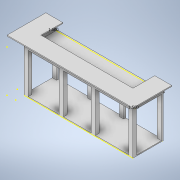
# Autodesk Inventor part: bardraft
Saved by Autodesk Inventor 2020 (Build 240168000, 168)
## iProperties
Created: 2020-07-25
Part Number: bardraft
Material: Generic
Document SubType Name: Modeling
Designer: al
Density: 1 g/cm^3
Appearance: Default
Author: al
Autodesk Inventor part; units mm, degrees
ref_plane "YZ Plane" through (0, 0, 0) normal (1, 0, 0) x (0, 1, 0)
ref_plane "XZ Plane" through (0, 0, 0) normal (0, 1, 0) x (-1, 0, 0)
ref_plane "XY Plane" through (0, 0, 0) normal (0, 0, 1) x (1, 0, 0)
sketch "Sketch1" plane through (0, 0, 0) normal (0, 0, 1) x (1, 0, 0)
  line L0 (0, 0) -> (0, 1092.2)
  line L1 (0, 1092.2) -> (812.8, 1092.2)
  line L2 (812.8, 1092.2) -> (812.8, 0)
  line L3 (812.8, 0) -> (0, 0)
  dimension "d0" = 1092.2
  dimension "d1" = 812.8
  constraints: 8 end point, 3 perpendicular, 1 vertical
  measures "d0" distance of L0.start L0.end
  measures "d1" distance of L0.end L1.end
extrude "Extrusion1" add sketch "Sketch1" along normal blind 2641.6
sketch "Sketch2" plane through (812.8, 0, 0) normal (1, 0, 0) x (0, 0, -1)
  line L0 (-2641.6, 1092.2) -> (-2641.6, 0) projected
  line L1 (-2641.6, 0) -> (-2463.8, 0)
  line L2 (0, 0) -> (-2641.6, 0) projected
  line L3 (-2463.8, 0) -> (-2463.8, 1073.15)
  line L4 (-2463.8, 1073.15) -> (-2641.6, 1073.15)
  line L5 (-2641.6, 1073.15) -> (-2641.6, 0)
  line L6 (0, 1092.2) -> (0, 0) projected
  line L7 (0, 0) -> (-177.8, 0)
  line L8 (-177.8, 0) -> (-177.8, 1073.15)
  line L9 (-177.8, 1073.15) -> (0, 1073.15)
  line L10 (0, 1073.15) -> (0, 0)
  dimension "d4" = 177.8
  dimension "d5" = 1073.15
  dimension "d6" = 177.8
  dimension "d7" = 1073.15
  constraints: 16 end point, 5 perpendicular, 2 point on line, 1 collinear
  measures "d4" distance of L0.end L1.end
  measures "d5" distance of L1.end L3.end
  measures "d6" distance of L2.start L7.end
  measures "d7" distance of L7.end L8.end
extrude "Extrusion2" cut sketch "Sketch2" against normal blind 2641.6
sketch "Sketch3" plane through (812.8, 0, 2463.8) normal (0, 0, 1) x (1, 0, 0)
  line L0 (0, 0) -> (-812.8, 0) projected
  line L1 (-812.8, 0) -> (-635, 0)
  line L2 (-635, 0) -> (-635, 1073.15)
  line L3 (-812.8, 1073.15) -> (0, 1073.15) projected
  line L4 (-812.8, 1073.15) -> (-812.8, 0)
  line L5 (-812.8, 1092.2) -> (-812.8, 1073.15) projected
  line L6 (-635, 1073.15) -> (-812.8, 1073.15)
  dimension "d10" = 177.8
  constraints: 8 end point, 2 point on line, 1 horizontal, 1 parallel, 1 perpendicular
  measures "d10" distance of L0.end L1.end
extrude "Extrusion3" cut sketch "Sketch3" against normal blind 2641.6
sketch "Sketch4" plane through (812.8, 0, 2463.8) normal (0, 0, 1) x (1, 0, 0)
  line L0 (0, 1073.15) -> (0, 0) projected
  line L1 (-635, 1073.15) -> (-635, 0) projected
  line L2 (-635, 0) -> (0, 0) projected
  line L3 (-635, 0) -> (-596.9, 0)
  line L4 (-596.9, 0) -> (-596.9, 19.05)
  line L5 (-596.9, 19.05) -> (-635, 19.05)
  line L6 (0, 0) -> (0, 1073.15) projected
  line L7 (0, 0) -> (0, 19.05)
  line L8 (0, 0) -> (-596.9, 0)
  line L9 (-596.9, 19.05) -> (-596.9, 1073.15)
  line L10 (-812.8, 1073.15) -> (0, 1073.15) projected
  line L11 (-635, 1073.15) -> (-596.9, 1073.15)
  line L12 (-635, 1073.15) -> (-635, 19.05)
  line L13 (-596.9, 19.05) -> (-558.8, 19.05)
  line L14 (-558.8, 19.05) -> (-558.8, 857.25)
  line L15 (-558.8, 857.25) -> (-596.9, 857.25)
  line L16 (-635, 0) -> (-635, 19.05)
  line L17 (-635, 19.05) -> (-25.4, 19.05)
  line L18 (-25.4, 19.05) -> (-25.4, 0)
  line L19 (-635, 0) -> (-25.4, 0)
  line L20 (-25.4, 19.05) -> (-63.5, 19.05)
  line L21 (-63.5, 19.05) -> (-63.5, 857.25)
  line L22 (-63.5, 857.25) -> (-25.4, 857.25)
  line L23 (-25.4, 857.25) -> (-25.4, 19.05)
  line L24 (-596.9, 857.25) -> (-596.9, 876.3)
  line L25 (-596.9, 876.3) -> (-25.4, 876.3)
  line L26 (-25.4, 876.3) -> (-25.4, 857.25)
  line L27 (-25.4, 857.25) -> (-596.9, 857.25)
  line L28 (-596.9, 876.3) -> (-596.9, 1092.2)
  line L29 (0, 1092.2) -> (-812.8, 1092.2) projected
  line L30 (-596.9, 1092.2) -> (0, 1092.2)
  line L31 (0, 1092.2) -> (0, 876.3)
  line L32 (-596.9, 876.3) -> (0, 876.3)
  line L33 (0, 876.3) -> (-25.4, 876.3)
  line L34 (-25.4, 876.3) -> (-25.4, 0)
  line L35 (0, 0) -> (-25.4, 0)
  line L36 (0, 0) -> (0, 876.3)
  point P0 (-812.8, 0)
  point P1 (-63.5, 857.25)
  point P2 (-25.4, 0)
  dimension "d13" = 635
  dimension "d15" = 19.05
  dimension "d16" = 38.1
  dimension "d17" = 838.2
  dimension "d18" = 609.6
  dimension "d19" = 38.1
  dimension "d20" = 838.2
  dimension "d21" = 19.05
  constraints: 62 end point, 14 perpendicular, 13 point on line, 6 collinear, 3 parallel, 1 horizontal, 1 vertical
  measures "d13" distance between parallel lines of L0 L1
  measures "d15" distance of L3.end L4.end
  measures "d16" distance of L4.end L13.end
  measures "d17" distance of L13.end L14.end
  measures "d18" distance of L5.end L17.end
  measures "d19" distance of L17.end L20.end
  measures "d20" distance of L20.end L21.end
  measures "d21" distance of L15.end L24.end
extrude "Extrusion4" cut sketch "Sketch4" against normal blind 2641.6 contours L0 L32 L25 L9 L10 | L0 L2 L18 L23 L26 L32 | L21 L17 L14 L27
sketch "Sketch6" plane through (0, 1092.2, 0) normal (0, 1, 0) x (1, 0, 0)
  line L0 (0, 0) -> (0, -2641.6) projected
  line L1 (0, 0) -> (0, -177.8)
  line L2 (177.8, -2463.8) -> (177.8, -177.8) projected
  line L3 (0, -177.8) -> (177.8, -177.8)
  line L4 (177.8, -177.8) -> (355.6, -177.8)
  line L5 (177.8, -177.8) -> (787.4, -177.8) projected
  line L6 (177.8, -177.8) -> (177.8, 0)
  line L7 (812.8, 0) -> (0, 0) projected
  line L8 (177.8, 0) -> (812.8, 0)
  line L9 (812.8, -2641.6) -> (812.8, 0) projected
  line L10 (812.8, 0) -> (812.8, -355.6)
  line L11 (812.8, -355.6) -> (355.6, -355.6)
  line L12 (812.8, -2641.6) -> (812.8, -2286)
  line L13 (812.8, -2286) -> (355.6, -2286)
  line L14 (355.6, -2286) -> (355.6, -355.6)
  line L15 (812.8, -355.6) -> (812.8, -2286)
  dimension "d25" = 177.8
  dimension "d26" = 177.8
  dimension "d27" = 355.6
  dimension "d28" = 457.2
  dimension "d29" = 355.6
  constraints: 22 end point, 4 perpendicular, 4 point on line, 2 vertical
  measures "d25" distance of L0.start L1.end
  measures "d26" distance of L2.end L4.end
  measures "d27" distance of L7.start L10.end
  measures "d28" distance of L10.end L11.end
  measures "d29" distance of L9.start L12.end
extrude "Extrusion5" cut sketch "Sketch6" against normal blind 25.4 contours L9 L13 L14 L11
sketch "Sketch7" plane through (215.9, 876.3, 2463.8) normal (0, 1, 0) x (1, 0, 0)
  line L0 (571.5, 0) -> (571.5, 2286) projected
  line L1 (0, 2286) -> (571.5, 2286)
  line L2 (571.5, 2286) -> (571.5, 2247.9)
  line L3 (0, 0) -> (0, 2286) projected
  line L4 (0, 2286) -> (0, 2247.9)
  line L5 (0, 2247.9) -> (571.5, 2247.9)
  line L6 (0, 0) -> (0, 38.1)
  line L7 (0, 38.1) -> (571.5, 38.1)
  line L8 (571.5, 0) -> (571.5, 38.1)
  line L9 (571.5, 0) -> (0, 0)
  point P0 (-215.9, 2463.8)
  point P1 (0, 38.1)
  dimension "d32" = 38.1
  dimension "d33" = 38.1
  dimension "d34" = 38.1
  constraints: 16 end point, 5 point on line, 4 perpendicular
  measures "d32" distance of L0.end L2.end
  measures "d33" distance of L1.start L4.end
  measures "d34" distance of L6.start L6.end
extrude "Extrusion6" add sketch "Sketch7" along normal blind 203.2 contours L9 L3 L7 L0 | L5 L3 L1 L0
sketch "Sketch8" plane through (177.8, 0, 177.8) normal (0, -1, 0) x (1, 0, 0)
  line L0 (609.6, 0) -> (609.6, 2286) projected
  line L1 (0, 2286) -> (0, 0) projected
  point P0 (-177.8, -177.8)
sketch "Sketch9" plane through (787.4, 0, 2463.8) normal (1, 0, 0) x (0, 0, -1)
  line L0 (38.1, 876.3) -> (2247.9, 876.3) projected
  line L1 (38.1, 876.3) -> (0, 876.3)
  line L2 (0, 1073.15) -> (0, 0) projected
  line L3 (0, 19.05) -> (0, 857.25) projected
  line L4 (0, 876.3) -> (0, 857.25)
  line L5 (0, 857.25) -> (2286, 857.25) projected
  line L6 (0, 857.25) -> (2286, 857.25)
  line L7 (2286, 857.25) -> (2286, 876.3)
  line L8 (2286, 0) -> (2286, 1073.15) projected
  line L9 (2286, 876.3) -> (0, 876.3)
  point P0 (2463.8, 0)
  dimension "d38" = 19.05
  dimension "d39" = 2286
  constraints: 10 end point, 3 point on line, 2 collinear, 1 horizontal, 1 perpendicular
  measures "d38" distance of L1.end L3.end
  measures "d39" distance of L3.end L5.end
extrude "Extrusion7" add sketch "Sketch9" along normal blind 25.4
sketch "Sketch10" plane through (215.9, 876.3, 215.9) normal (0, 1, 0) x (1, 0, 0)
  line L0 (596.9, 38.1) -> (596.9, -2247.9) projected
  line L1 (0, -2209.8) -> (0, 0) projected
  point P0 (-215.9, 215.9)
sketch "Sketch11" plane through (215.9, 876.3, 215.9) normal (1, 0, 0) x (0, 0, -1)
  line L0 (-2209.8, 0) -> (-2209.8, 196.85)
  line L1 (-2247.9, 196.85) -> (38.1, 196.85) projected
  line L2 (0, 0) -> (0, 196.85) projected
  line L3 (0, 196.85) -> (-2209.8, 196.85)
  line L4 (-2209.8, 0) -> (0, 0) projected
  line L5 (-2209.8, 0) -> (0, 0)
  line L6 (0, 0) -> (0, 196.85)
  line L7 (0, 0) -> (0, 196.85)
  point P0 (215.9, -876.3)
  constraints: 10 end point, 2 perpendicular, 1 collinear, 1 horizontal, 1 point on line, 1 vertical
sketch "Sketch12" plane through (787.4, 0, 2463.8) normal (1, 0, 0) x (0, 0, -1)
  line L0 (0, 0) -> (0, 857.25) projected
  line L1 (0, 857.25) -> (2286, 857.25) projected
  line L2 (0, 0) -> (0, 857.25)
  line L3 (0, 857.25) -> (2286, 857.25)
  line L4 (2286, 857.25) -> (2286, 0) projected
  line L5 (2286, 857.25) -> (2286, 0)
  line L6 (2286, 0) -> (0, 0)
  point P0 (2463.8, 0)
  constraints: 8 end point, 4 perpendicular
extrude "Extrusion8" add sketch "Sketch12" along normal blind 25.4
sketch "Sketch13" plane through (787.4, 876.3, 2463.8) normal (1, 0, 0) x (0, 0, -1)
  line L0 (38.1, 0) -> (38.1, 196.85) projected
  line L1 (0, 196.85) -> (38.1, 196.85)
  line L2 (38.1, 196.85) -> (38.1, 0)
  line L3 (38.1, 0) -> (0, 0)
  line L4 (0, 0) -> (0, 196.85)
  point P0 (2463.8, -876.3)
  constraints: 8 end point, 2 parallel, 1 horizontal, 1 perpendicular
extrude "Extrusion9" add sketch "Sketch13" along normal blind 25.4
sketch "Sketch14" plane through (787.4, 876.3, 177.8) normal (1, 0, 0) x (0, 0, -1)
  line L0 (-38.1, 0) -> (-38.1, 196.85) projected
  line L1 (0, 196.85) -> (0, 0) projected
  line L2 (-38.1, 196.85) -> (0, 196.85)
  line L3 (0, 196.85) -> (0, 0)
  line L4 (0, 0) -> (-38.1, 0)
  line L5 (-38.1, 0) -> (-38.1, 196.85)
  point P0 (177.8, -876.3)
  constraints: 8 end point, 2 parallel, 1 horizontal, 1 perpendicular
extrude "Extrusion10" add sketch "Sketch14" along normal blind 25.4
sketch "Sketch15" plane through (812.8, 0, 2463.8) normal (1, 0, 0) x (0, 0, -1)
  line L0 (38.1, 876.3) -> (2247.9, 876.3) projected
  line L1 (0, 857.25) -> (2286, 857.25) projected
  line L2 (38.1, 876.3) -> (0, 876.3)
  line L3 (0, 876.3) -> (0, 857.25)
  line L4 (0, 857.25) -> (2286, 857.25)
  line L5 (2286, 0) -> (2286, 1073.15) projected
  line L6 (2286, 857.25) -> (2286, 876.3)
  line L7 (0, 876.3) -> (2286, 876.3)
  point P0 (2463.8, 0)
  constraints: 10 end point, 3 perpendicular, 2 point on line, 1 horizontal
extrude "Extrusion11" add sketch "Sketch15" along normal blind 25.4
sketch "Sketch16" plane through (215.9, 876.3, 215.9) normal (0, 1, 0) x (1, 0, 0)
  line L0 (0, -2209.8) -> (596.9, -2209.8) projected
  line L1 (0, -2209.8) -> (38.1, -2209.8)
  point P0 (-215.9, 215.9)
  dimension "d51" = 38.1
  constraints: 2 end point, 1 point on line
  measures "d51" distance of L0.start L1.end
sketch "Sketch17" plane through (215.9, 876.3, 215.9) normal (0, 1, 0) x (1, 0, 0)
  line L0 (0, -2209.8) -> (0, 0) projected
  line L1 (0, -2209.8) -> (38.1, -2209.8)
  line L2 (38.1, -2247.9) -> (38.1, 38.1) projected
  line L3 (38.1, -2209.8) -> (38.1, 0)
  line L4 (596.9, 0) -> (0, 0) projected
  line L5 (0, 0) -> (38.1, 4.2904)
  line L6 (38.1, 0) -> (0, 0)
  line L7 (0, 0) -> (0, -2209.8)
  point P0 (-215.9, 215.9)
  dimension "d52" = 38.1
  constraints: 10 end point, 3 point on line, 1 collinear, 1 horizontal, 1 perpendicular
  measures "d52" distance of L0.start L1.end
extrude "Extrusion12" cut sketch "Sketch17" against normal blind 19.05 contours L0 L4 L2 L1
sketch "Sketch18" plane through (812.8, 0, 177.8) normal (0, 0, -1) x (-1, 0, 0)
  line L0 (558.8, 857.25) -> (63.5, 857.25) projected
  line L1 (63.5, 857.25) -> (38.1, 857.25)
  line L2 (38.1, 857.25) -> (38.1, 19.05)
  line L3 (38.1, 19.05) -> (63.5, 19.05)
  line L4 (63.5, 19.05) -> (63.5, 857.25) projected
  line L5 (63.5, 19.05) -> (63.5, 857.25)
  point P0 (812.8, 0)
  dimension "d58" = 25.4
  dimension "d59" = 838.2
  constraints: 8 end point, 2 perpendicular, 1 collinear, 1 horizontal
  measures "d58" distance of L0.end L1.end
  measures "d59" distance of L1.end L2.end
extrude "Extrusion13" cut sketch "Sketch18" against normal blind 3810
sketch "Sketch21" plane through (254, 19.05, 2463.8) normal (1, 0, 0) x (0, 0, -1)
  line L0 (0, 0) -> (88.9, 0)
  line L1 (88.9, 0) -> (88.9, 838.2)
  line L2 (38.1, 838.2) -> (2247.9, 838.2) projected
  line L3 (88.9, 838.2) -> (0, 838.2)
  line L4 (0, 838.2) -> (0, 0)
  line L5 (88.9, 0) -> (787.4, 0)
  line L6 (0, 0) -> (2286, 0) projected
  line L7 (787.4, 0) -> (787.4, 838.2)
  line L8 (787.4, 838.2) -> (876.3, 838.2)
  line L9 (876.3, 838.2) -> (876.3, 0)
  line L10 (88.9, 838.2) -> (787.4, 838.2)
  line L11 (38.1, 838.2) -> (2247.9, 838.2) projected
  line L12 (876.3, 0) -> (1460.5, 0)
  line L13 (1460.5, 0) -> (1460.5, 838.2)
  line L14 (1460.5, 838.2) -> (1549.4, 838.2)
  line L15 (1549.4, 838.2) -> (1549.4, 0)
  line L16 (1549.4, 0) -> (1460.5, 0)
  line L17 (2286, 838.2) -> (2286, 0) projected
  line L18 (2286, 0) -> (2197.1, 0)
  line L19 (2197.1, 0) -> (2197.1, 838.2)
  line L20 (2197.1, 838.2) -> (1549.4, 838.2)
  line L21 (2197.1, 0) -> (1549.4, 0)
  line L22 (0, -19.05) -> (2286, -19.05) projected
  point P0 (2463.8, -19.05)
  point P1 (876.3, 0)
  dimension "d72" = 88.9
  dimension "d73" = 698.5
  dimension "d74" = 838.2
  dimension "d75" = 88.9
  dimension "d76" = 584.2
  dimension "d77" = 838.2
  dimension "d78" = 88.9
  dimension "d79" = 838.2
  dimension "d80" = 88.9
  dimension "d81" = 838.2
  constraints: 36 end point, 11 point on line, 2 collinear, 2 horizontal, 2 perpendicular, 1 parallel, 1 vertical
  measures "d72" distance of L0.start L0.end
  measures "d73" distance of L0.end L5.end
  measures "d74" distance of L5.end L7.end
  measures "d75" distance of L7.end L8.end
  measures "d76" distance of L9.end L12.end
  measures "d77" distance of L12.end L13.end
  measures "d78" distance of L13.end L14.end
  measures "d79" distance of L14.end L15.end
  measures "d80" distance of L6.end L18.end
  measures "d81" distance of L18.end L19.end
extrude "Extrusion14" cut sketch "Sketch21" along normal through all both and the other way through all contours L1 L2 L7 L5 | L9 L2 L13 L6 | L15 L2 L19 L6
sketch "Sketch22" plane through (812.8, 0, 177.8) normal (0, 0, -1) x (-1, 0, 0)
  line L0 (0, 876.3) -> (558.8, 876.3) projected
  line L1 (0, 876.3) -> (38.1, 876.3)
  point P0 (812.8, 0)
  dimension "d84" = 38.1
  constraints: 2 end point, 1 point on line
  measures "d84" distance of L0.start L1.end
body "Solid1"
